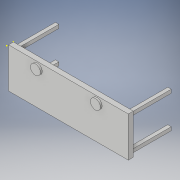
# Autodesk Inventor part: Master-workspace
Saved by Autodesk Inventor 2019 (Build 230136000, 136)
## iProperties
Created: 2019-11-01
Part Number: Master-workspace
Material: Generic
Document SubType Name: Modeling
Designer: Nikol
Density: 1 g/cm^3
Appearance: Default
Author: Nikol
Autodesk Inventor part; units mm, degrees
ref_plane "YZ Plane" through (0, 0, 0) normal (1, 0, 0) x (0, 1, 0)
ref_plane "XZ Plane" through (0, 0, 0) normal (0, 1, 0) x (-1, 0, 0)
ref_plane "XY Plane" through (0, 0, 0) normal (0, 0, 1) x (1, 0, 0)
sketch "Sketch1" plane through (0, 0, 0) normal (0, 0, 1) x (1, 0, 0)
  line L0 (0, 0) -> (2400, 0)
  line L1 (2400, 0) -> (2400, -800)
  line L2 (2400, -800) -> (0, -800)
  line L3 (0, -800) -> (0, 0)
  line L4 (0, 0) -> (575, 0)
  line L5 (575, 0) -> (575, -125)
  line L6 (0, 0) -> (1775, 0)
  line L7 (1775, 0) -> (1775, -125)
  circle A0 centre (575, -125) radius 100
  circle A1 centre (1775, -125) radius 100
  dimension "d0" = 2400
  dimension "d1" = 800
  dimension "d2" = 575
  dimension "d3" = 125
  dimension "d4" = 1775
  dimension "d5" = 200
  constraints: 16 end point, 3 perpendicular, 2 centre point, 2 coincident, 2 parallel, 2 point on line, 1 horizontal
  measures "d0" distance of L1.end L2.end
  measures "d1" distance of L0.end L1.end
  measures "d2" distance of L0.start L4.end
  measures "d3" distance of L4.end L5.end
  measures "d4" distance of L0.start L6.end
  measures "d5" diameter of A0
extrude "Extrusion1" add sketch "Sketch1" along normal blind 35 contours A1 | A0
extrude "Extrusion2" add sketch "Sketch1" against normal blind 100
sketch "Sketch2" plane through (575, -125, 35) normal (0, 0, 1) x (1, 0, 0)
  point P0 (-575, 125)
extrude "Extrusion3" add sketch "Sketch1" against normal blind 100 contours A0
extrude "Extrusion4" add sketch "Sketch1" against normal blind 100 contours A1
sketch "Sketch3" plane through (0, 0, -100) normal (0, 0, -1) x (-1, 0, 0)
  point P0 (0, 0)
sketch "Sketch4" plane through (0, 0, -100) normal (0, 0, -1) x (-1, 0, 0)
  line L0 (0, 0) -> (-2400, 0) projected
  line L1 (0, 0) -> (0, -40)
  line L2 (0, -800) -> (0, 0) projected
  line L3 (0, -40) -> (-40, -40)
  line L4 (-40, -40) -> (-110, -40)
  line L5 (-110, -40) -> (-110, -110)
  line L6 (-110, -110) -> (-40, -110)
  line L7 (-40, -110) -> (-40, -40)
  line L8 (-2400, -800) -> (0, -800) projected
  line L9 (0, -800) -> (-40, -800)
  line L10 (0, -760) -> (0, -800)
  line L11 (-40, -760) -> (-110, -760)
  line L12 (-110, -760) -> (-110, -690)
  line L13 (-110, -690) -> (-40, -690)
  line L14 (-40, -690) -> (-40, -760)
  line L15 (-2400, 0) -> (-2400, -800) projected
  line L16 (-2400, 0) -> (-2400, -40)
  line L17 (-2400, -40) -> (-2360, -40)
  line L18 (-2400, -800) -> (-2400, -760)
  line L19 (-2400, -760) -> (-2360, -760)
  line L20 (-2360, -40) -> (-2290, -40)
  line L21 (-2290, -40) -> (-2290, -110)
  line L22 (-2290, -110) -> (-2360, -110)
  line L23 (-2360, -110) -> (-2360, -40)
  line L24 (-2360, -760) -> (-2290, -760)
  line L25 (-2290, -760) -> (-2290, -690)
  line L26 (-2290, -690) -> (-2360, -690)
  line L27 (-2360, -690) -> (-2360, -760)
  dimension "d14" = 40
  dimension "d15" = 40
  dimension "d16" = 70
  dimension "d17" = 70
  dimension "d18" = 40
  dimension "d19" = 40
  dimension "d20" = 70
  dimension "d21" = 70
  dimension "d22" = 40
  dimension "d23" = 40
  dimension "d24" = 70
  dimension "d25" = 70
  dimension "d26" = 70
  dimension "d27" = 70
  constraints: 48 end point, 8 parallel, 6 horizontal, 6 perpendicular, 3 point on line
  measures "d14" distance of L0.start L1.end
  measures "d15" distance of L1.end L3.end
  measures "d16" distance of L6.end L5.end
  measures "d17" distance of L5.end L4.end
  measures "d18" distance of L11.start L10.start
  measures "d19" distance of L9.end L11.start
  measures "d20" distance of L12.end L13.end
  measures "d21" distance of L11.end L12.end
  measures "d22" distance of L0.end L16.end
  measures "d23" distance of L16.end L17.end
  measures "d24" distance of L21.end L22.end
  measures "d25" distance of L20.end L21.end
  measures "d26" distance of L26.end L25.end
  measures "d27" distance of L25.end L24.end
extrude "Extrusion5" add sketch "Sketch4" along normal blind 800 contours L20 L21 L22 L23 | L27 L26 L25 L24 | L7 L6 L5 L4 | L11 L12 L13 L14
body "Solid1"
